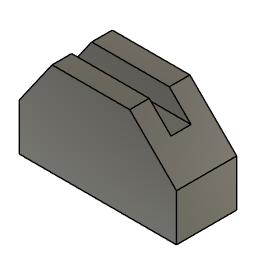
3D Plancha 6 (Autodesk Fusion 360 design; units mm, degrees)
Autodesk Fusion 360 part; units mm, degrees
sketch "Boceto1" plane through (0, 0, 0) normal (0, 0, 1) x (1, 0, 0)
sketch "Boceto2" plane through (0, 0, 0) normal (0, 0, 1) x (1, 0, 0)
box "CajaPrimitiva1" add length 18 width 47 height 28 placed x (0, -1, 0) y (1, 0, 0) z (0, 0, 1) at (0, 0, 0) makes body 1
copy_body "CopiarPegarCuerpos2" bodies 1 makes body 2
move_body "Desplazar2" bodies 2 to x (1, 0, 0) y (0, 1, 0) z (0, 0, 1) at (0, 0, 0)
move_body "Desplazar3" bodies 2 to x (1, 0, 0) y (0, 1, 0) z (0, 0, 1) at (0, 0, 30)
move_body "Desplazar6" bodies 2 to x (1, 0, 0) y (0, 1, 0) z (0, 0, 1) at (47, 0, 13)
move_body "Alinear1" bodies 2 to x (1, 0, 0) y (0, 1, 0) z (0, 0, 1) at (0, 0, -29)
move_body "Desplazar7" bodies 2 to x (0.707107, 0, 0.707107) y (0, 1, 0) z (-0.707107, 0, 0.707107) at (23.6655, 0, -29.1335)
combine "Combinar1" operation cut target body 1 tool bodies 2
copy_body "CopiarPegarCuerpos3" bodies 1 makes body 3
move_body "Desplazar8" bodies 3 to x (1, 0, 0) y (0, 1, 0) z (0, 0, 1) at (0, 0, 0)
move_body "Desplazar9" bodies 3 to x (-1, 0, 0) y (0, -1, 0) z (0, 0, 1) at (-2, -26, 21)
move_body "Desplazar10" bodies 3 to x (1, 0, 0) y (0, 1, 0) z (0, 0, 1) at (-15, 0, 0)
move_body "Alinear2" bodies 3 to x (1, 0, 0) y (0, 1, 0) z (0, 0, 1) at (17, 8, -7)
move_body "Desplazar11" bodies 3 to x (0.819152, 0, -0.573576) y (0, 1, 0) z (0.573576, 0, 0.819152) at (-8.0301, 0, 2.5319)
combine "Combinar2" operation cut target body 1 tool bodies 3
box "CajaPrimitiva2" add length 47 width 6 height 7 placed x (0, -1, 0) y (1, 0, 0) z (0, 0, 1) at (0, -50, 0) separate body makes body 4
move_body "Desplazar12" bodies 4 to x (0, -1, 0) y (0.996195, 0, -0.087156) z (0.087156, 0, 0.996195) at (97.6268, -2.854, 16.5543)
move_body "Desplazar13" bodies 4 to x (1, 0, 0) y (0, 1, 0) z (0, 0, 1) at (0, 15, 0)
move_body "Desplazar14" bodies 4 to x (1, 0, 0) y (0, 1, 0) z (0, 0, 1) at (0, -18.3, 0)
move_face "MoveFace1" to x (0.996195, 0, -0.087156) y (0, 1, 0) z (0.087156, 0, 0.996195) at (-1.9632, 0, 4.0085) 1 faces at (16.8063, -12.154, 25.9674) on bodies 4
move_body "Desplazar15" bodies 4 to x (0.996195, 0, 0.087156) y (0, 1, 0) z (-0.087156, 0, 0.996195) at (1.8264, 0, -0.0072)
move_body "Desplazar16" bodies 4 to x (1, 0, 0) y (0, 1, 0) z (0, 0, 1) at (0, 0, -4)
move_body "Desplazar17" bodies 4 to x (1, 0, 0) y (0, 1, 0) z (0, 0, 1) at (0, 0, 0.5)
combine "Combinar3" operation cut target body 1 tool bodies 4
